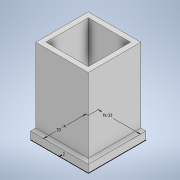
# Autodesk Inventor part: single
Saved by Autodesk Inventor 2022 (Build 260153000, 153)
## iProperties
Created: 2021-10-08
Part Number: single
Material: Generic
Document SubType Name: Modeling
Designer: dangl
Density: 1 g/cm^3
Appearance: Default
Author: dangl
Autodesk Inventor part; units mm, degrees
ref_plane "YZ Plane" through (0, 0, 0) normal (1, 0, 0) x (0, 1, 0)
ref_plane "XZ Plane" through (0, 0, 0) normal (0, 1, 0) x (-1, 0, 0)
ref_plane "XY Plane" through (0, 0, 0) normal (0, 0, 1) x (1, 0, 0)
sketch "Sketch1" plane through (0, 0, 0) normal (0, 1, 0) x (-1, 0, 0)
  line L0 (0, 0) -> (33, 0)
  line L1 (33, 0) -> (33, -33)
  line L2 (33, -33) -> (0, -33)
  line L3 (0, -33) -> (0, 0)
  line L4 (0, -33) -> (0, 0)
  line L5 (37, -37) -> (37, 4)
  line L6 (37, 4) -> (-4, 4)
  line L7 (-4, 4) -> (-4, -37)
  line L8 (-4, -37) -> (37, -37)
  line L9 (-6, 6) -> (39, 6)
  line L10 (39, 6) -> (39, -39)
  line L11 (39, -39) -> (-6, -39)
  line L12 (-6, -39) -> (-6, 6)
  point P0 (0, -33)
  point P1 (0, -37)
  point P2 (0, 4)
  dimension "d0" = 33
  dimension "d1" = 33
  dimension "d5" = 4
  dimension "d10" = 2
  constraints: 26 end point, 6 parallel, 3 perpendicular, 1 horizontal, 1 point on line, 6 other
  measures "d0" distance of L0.end L1.end
  measures "d1" distance of L2.end L1.end
  measures "d5" distance between parallel lines of L1 L5
  measures "d10" distance between parallel lines of L6 L9
extrude "Extrusion1" add sketch "Sketch1" along normal blind 6 contours L0 L1 L2 L3 | L8 L7 L6 L5 | L9 L10 L11 L12
extrude "Extrusion3" add sketch "Sketch1" along normal blind 66 contours L8 L7 L6 L5
chamfer "Chamfer3" distance 2 angle 45 4 edges at (-16.5, 6, 4) (4, 6, -16.5) (-16.5, 6, -37) (-37, 6, -16.5)
equation "\"d1\" = d0"
body "Solid1"
